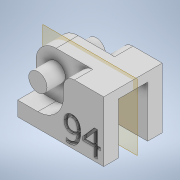
# Autodesk Inventor part: 1번부품
Saved by Autodesk Inventor 2022 (Build 260153000, 153)
## iProperties
Created: 2021-09-11
Part Number: 1번부품
Material: 일반
Document SubType Name: Modeling
Designer: 서울공업고등학교
Density: 1 g/cm^3
Appearance: 기본값
Author: 서울공업고등학교
Autodesk Inventor part; units mm, degrees
ref_plane "YZ Plane" through (0, 0, 0) normal (1, 0, 0) x (0, 1, 0)
ref_plane "XZ Plane" through (0, 0, 0) normal (0, 1, 0) x (-1, 0, 0)
ref_plane "XY Plane" through (0, 0, 0) normal (0, 0, 1) x (1, 0, 0)
sketch "스케치1" plane through (0, 0, 0) normal (0, 0, 1) x (1, 0, 0)
  line L0 (-11.75, 8.25) -> (11.75, 8.25)
  line L1 (11.75, 8.25) -> (11.75, -8.25)
  line L2 (11.75, -8.25) -> (-11.75, -8.25)
  line L3 (-11.75, -8.25) -> (-11.75, 8.25)
  line L4 (-11.75, 8.25) -> (11.75, -8.25) construction
  line L5 (11.75, 8.25) -> (-11.75, -8.25) construction
  line L6 (-11.75, -4.25) -> (0.75, -4.25)
  line L7 (0.75, -4.25) -> (0.75, 8.25)
  circle A0 centre (-6.25, 2.75) radius 2.5
  point P0 (0, 0)
  dimension "d0" = 23.5
  dimension "d1" = 16.5
  dimension "d3" = 4
  dimension "d4" = 12.5
  dimension "d5" = 5
  dimension "d6" = 11
  dimension "d7" = 18
  constraints: 16 end point, 2 horizontal, 2 midpoint, 2 parallel, 2 perpendicular, 2 point on line, 1 centre point
  measures "d0" distance of L1.end L2.end
  measures "d1" distance of L0.end L1.end
  measures "d3" distance between parallel lines of L6 L2
  measures "d4" distance of L6.start L6.end
  measures "d5" diameter of A0
  measures "d6" distance from line of A0.centre L2
  measures "d7" distance from line of L1 A0.centre
extrude "돌출1" add sketch "스케치1" along normal mid plane 16 contours L0 L1 L2 L3 L6 L7 | A0
extrude "돌출2" add sketch "스케치1" along normal mid plane 6 contours L0 L7 L6 L3
ref_plane "작업 평면1" through (0, 0, 0) normal (0, 0, 1) x (1, 0, 0)
sketch "스케치2" plane through (0, 0, 0) normal (0, 0, 1) x (1, 0, 0)
  line L0 (11.75, 8.25) -> (11.75, -8.25) projected
  line L1 (11.75, 5.75) -> (-3.25, -8.25)
  line L2 (-11.75, -8.25) -> (-11.75, -4.25) projected
  line L3 (11.75, -8.25) -> (-11.75, -8.25) projected
  point P0 (0, 0)
  dimension "d12" = 2.5
  dimension "d13" = 8.5
  dimension "d14" = 0
  constraints: 2 end point, 1 point on line
  measures "d12" distance of L0.start L1.start
  measures "d13" distance from line of L2 L1.end
  measures "d14" distance from line of L3 L1.end
extrude "돌출3" cut sketch "스케치2" along normal mid plane 8
fillet "모깎기1" radius 3 2 edges at (0.75, 8.25, 5.5) (0.75, 8.25, -5.5)
fillet "모깎기2" radius 5.5 1 edges at (-11.75, 8.25, 0)
fillet "모깎기3" radius 7 2 edges at (0.75, -4.25, 5.5) (0.75, -4.25, -5.5)
sketch "스케치3" plane through (0, 0, 8) normal (0, 0, 1) x (1, 0, 0)
  line L0 (0.5954, -0.2053) -> (15.6035, -0.2053) construction
  line L1 (15.6035, -0.2053) -> (15.6035, -10.6024) construction
  line L2 (15.6035, -10.6024) -> (0.5954, -10.6024) construction
  line L3 (0.5954, -10.6024) -> (0.5954, -0.2053) construction
  spline S0 degree 2 poles (0.9131, -2.6219) (0.9131, -2.083) (1.2648, -1.1867) (1.5711, -0.8633) knots 0 0 0 1 2 2 2
  spline S1 degree 2 poles (1.5711, -0.8633) (1.8604, -0.5513) (2.7056, -0.2053) (3.1368, -0.2053) knots 0 0 0 1 2 2 2
  spline S2 degree 2 poles (3.1368, -0.2053) (3.6189, -0.2053) (4.4017, -0.5287) (4.691, -0.835) knots 0 0 0 1 2 2 2
  spline S3 degree 2 poles (4.691, -0.835) (5.0541, -1.2207) (5.4512, -2.4687) (5.4512, -3.4274) knots 0 0 0 1 2 2 2
  spline S4 degree 2 poles (5.4512, -3.4274) (5.4512, -4.2953) (5.0598, -5.8496) (4.6797, -6.3658) knots 0 0 0 1 2 2 2
  spline S5 degree 2 poles (4.6797, -6.3658) (4.2769, -6.9103) (3.1424, -7.4833) (2.3142, -7.4833) knots 0 0 0 1 2 2 2
  spline S6 degree 2 poles (2.3142, -7.4833) (2.127, -7.4833) (1.7016, -7.4436) (1.5201, -7.3868) knots 0 0 0 1 2 2 2
  line L4 (1.5201, -7.3868) -> (1.5201, -6.4849)
  line L5 (1.5201, -6.4849) -> (1.5654, -6.4849)
  spline S7 degree 2 poles (1.5654, -6.4849) (1.6846, -6.553) (2.1838, -6.6721) (2.439, -6.6721) knots 0 0 0 1 2 2 2
  spline S8 degree 2 poles (2.439, -6.6721) (3.358, -6.6721) (4.4074, -5.4582) (4.4812, -4.335) knots 0 0 0 1 2 2 2
  spline S9 degree 2 poles (4.4812, -4.335) (4.1068, -4.5902) (3.4261, -4.8228) (3.0233, -4.8228) knots 0 0 0 1 2 2 2
  spline S10 degree 2 poles (3.0233, -4.8228) (2.6376, -4.8228) (1.9966, -4.6526) (1.6732, -4.4087) knots 0 0 0 1 2 2 2
  spline S11 degree 2 poles (1.6732, -4.4087) (1.2988, -4.1194) (0.9131, -3.2402) (0.9131, -2.6219) knots 0 0 0 1 2 2 2
  spline S12 degree 2 poles (4.5039, -3.2175) (4.5039, -2.5084) (4.2429, -1.6121) (4.0103, -1.3682) knots 0 0 0 1 2 2 2
  spline S13 degree 2 poles (4.0103, -1.3682) (3.8061, -1.1413) (3.3807, -0.9711) (3.1311, -0.9711) knots 0 0 0 1 2 2 2
  spline S14 degree 2 poles (3.1311, -0.9711) (2.5525, -0.9711) (1.8661, -1.7993) (1.8661, -2.5821) knots 0 0 0 1 2 2 2
  spline S15 degree 2 poles (1.8661, -2.5821) (1.8661, -3.0246) (2.093, -3.5975) (2.3426, -3.8018) knots 0 0 0 1 2 2 2
  spline S16 degree 2 poles (2.3426, -3.8018) (2.5241, -3.9492) (2.9722, -4.0457) (3.2332, -4.0457) knots 0 0 0 1 2 2 2
  spline S17 degree 2 poles (3.2332, -4.0457) (3.5338, -4.0457) (4.2259, -3.8358) (4.4868, -3.6599) knots 0 0 0 1 2 2 2
  spline S18 degree 2 poles (4.4868, -3.6599) (4.4925, -3.5919) (4.5039, -3.3593) (4.5039, -3.2175) knots 0 0 0 1 2 2 2
  line L6 (10.8628, -4.9419) -> (10.029, -4.9419)
  line L7 (10.029, -4.9419) -> (10.029, -7.3471)
  line L8 (10.029, -7.3471) -> (9.127, -7.3471)
  line L9 (9.127, -7.3471) -> (9.127, -4.9419)
  line L10 (9.127, -4.9419) -> (6.0355, -4.9419)
  line L11 (6.0355, -4.9419) -> (6.0355, -3.9549)
  line L12 (6.0355, -3.9549) -> (9.1667, -0.3471)
  line L13 (9.1667, -0.3471) -> (10.029, -0.3471)
  line L14 (10.029, -0.3471) -> (10.029, -4.1875)
  line L15 (10.029, -4.1875) -> (10.8628, -4.1875)
  line L16 (10.8628, -4.1875) -> (10.8628, -4.9419)
  line L17 (9.127, -4.1875) -> (9.127, -1.4533)
  line L18 (9.127, -1.4533) -> (6.7729, -4.1875)
  line L19 (6.7729, -4.1875) -> (9.127, -4.1875)
  point P0 (0, 0)
  constraints: 2 other
extrude "돌출4" cut sketch "스케치3" against normal blind 1
